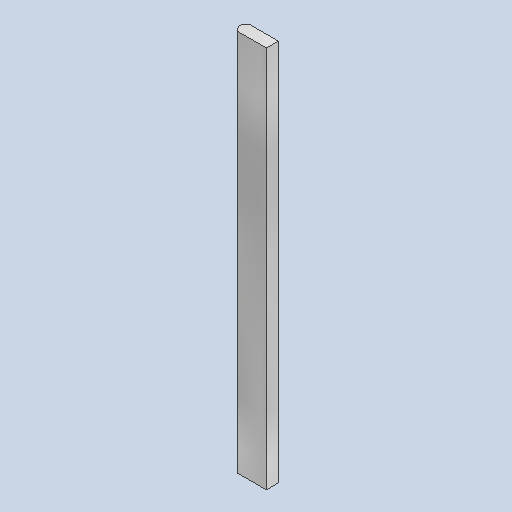
# Autodesk Inventor part: 窗側柱
Saved by Autodesk Inventor 2024.2 (Build 282272000, 272)
## iProperties
Created: 2024-06-01
Part Number: 窗側柱
Material: 一般
Document SubType Name: Modeling
Designer: User
Density: 1 g/cm^3
Appearance: 預設
Author: User
Autodesk Inventor part; units mm, degrees
ref_plane "YZ Plane" through (0, 0, 0) normal (1, 0, 0) x (0, 1, 0)
ref_plane "XZ Plane" through (0, 0, 0) normal (0, 1, 0) x (-1, 0, 0)
ref_plane "XY Plane" through (0, 0, 0) normal (0, 0, 1) x (1, 0, 0)
sketch "草圖1" plane through (0, 0, 0) normal (0, 1, 0) x (-1, 0, 0)
  line L0 (0, 0) -> (0, -0.25)
  line L1 (0, 0) -> (0, -0.25)
  line L2 (0, -0.25) -> (-0.6, -0.25)
  line L3 (-0.6, -0.25) -> (-0.6, 0)
  line L4 (-0.6, 0) -> (0, 0)
  line L5 (0, 0) -> (0.125, -0.125)
  line L6 (0.125, -0.125) -> (0, -0.25)
  dimension "d0" = 0.25
  dimension "d1" = 0.6
  dimension "d2" = 45
  constraints: 14 end point, 3 equal length, 2 perpendicular, 1 vertical
  measures "d0" distance of L0.start L0.end
  measures "d1" distance of L0.end L2.end
  measures "d2" angle of L0 L6
extrude "擠出1" add sketch "草圖1" along normal blind 8
fillet "圓角1" radius 0.1 1 edges at (-0.125, 4, -0.125)
